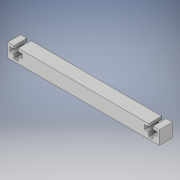
# Autodesk Inventor part: horzntalconnection
Saved by Autodesk Inventor 2017 (Build 210142000, 142)
## iProperties
Created: 2017-11-22
Part Number: horzntalconnection
Material: Generic
Document SubType Name: Modeling
Designer: build
Density: 1 g/cm^3
Appearance: Default
Author: build
Autodesk Inventor part; units mm, degrees
ref_plane "YZ Plane" through (0, 0, 0) normal (1, 0, 0) x (0, 1, 0)
ref_plane "XZ Plane" through (0, 0, 0) normal (0, 1, 0) x (-1, 0, 0)
ref_plane "XY Plane" through (0, 0, 0) normal (0, 0, 1) x (1, 0, 0)
sketch "Sketch1" plane through (0, 0, 0) normal (1, 0, 0) x (0, 1, 0)
  line L0 (0, 0) -> (16.383, 0)
  line L1 (16.383, 0) -> (16.383, -15.875)
  line L2 (16.383, -15.875) -> (0, -15.875)
  line L3 (0, -15.875) -> (0, 0)
  dimension "d0" = 16.383
  dimension "d1" = 15.875
  constraints: 8 end point, 2 parallel, 1 horizontal, 1 perpendicular
  measures "d0" distance of L0.start L0.end
  measures "d1" distance of L0.end L1.end
extrude "Extrusion1" add sketch "Sketch1" along normal blind 184.15
sketch "Sketch2" plane through (0, 0, -15.875) normal (0, 0, -1) x (-1, 0, 0)
  line L0 (-184.15, 16.383) -> (-184.15, 0) projected
  line L1 (-184.15, 16.383) -> (-176.53, 16.383)
  line L2 (0, 16.383) -> (-184.15, 16.383) projected
  line L3 (-176.53, 16.383) -> (-176.53, 13.081)
  line L4 (-176.53, 13.081) -> (-181.61, 13.081)
  line L5 (-181.61, 13.081) -> (-181.61, 8.001)
  line L6 (-181.61, 8.001) -> (-176.53, 8.001)
  line L7 (-176.53, 8.001) -> (-176.53, 2.921)
  line L8 (-176.53, 2.921) -> (-171.45, 2.921)
  line L9 (-171.45, 2.921) -> (-171.45, 8.001)
  line L10 (-171.45, 8.001) -> (-166.37, 8.001)
  line L11 (-166.37, 8.001) -> (-166.37, 13.081)
  line L12 (-166.37, 13.081) -> (-171.45, 13.081)
  line L13 (-171.45, 16.383) -> (-171.45, 13.081)
  line L14 (0, 16.383) -> (-7.62, 16.383)
  line L15 (-7.62, 16.383) -> (-7.62, 13.081)
  line L16 (-7.62, 13.081) -> (-2.54, 13.081)
  line L17 (-2.54, 13.081) -> (-2.54, 8.001)
  line L18 (-2.54, 8.001) -> (-7.62, 8.001)
  line L19 (-7.62, 8.001) -> (-7.62, 2.921)
  line L20 (-7.62, 2.921) -> (-12.7, 2.921)
  line L21 (-12.7, 2.921) -> (-12.7, 8.001)
  line L22 (-12.7, 8.001) -> (-17.78, 8.001)
  line L23 (-17.78, 8.001) -> (-17.78, 13.081)
  line L24 (-17.78, 13.081) -> (-12.7, 13.081)
  line L25 (-12.7, 13.081) -> (-12.7, 16.383)
  point P0 (0, 0)
  dimension "d4" = 7.62
  dimension "d5" = 3.302
  dimension "d6" = 5.08
  dimension "d7" = 5.08
  dimension "d8" = 5.08
  dimension "d9" = 5.08
  dimension "d10" = 5.08
  dimension "d11" = 7.62
  dimension "d12" = 3.302
  dimension "d13" = 5.08
  dimension "d14" = 5.08
  dimension "d15" = 5.08
  constraints: 48 end point, 14 perpendicular, 13 point on line, 3 vertical, 1 horizontal, 1 parallel
  measures "d4" distance of L0.start L1.end
  measures "d5" distance of L1.end L3.end
  measures "d6" distance of L3.end L4.end
  measures "d7" distance of L4.end L5.end
  measures "d8" distance of L6.end L7.end
  measures "d9" distance of L7.end L8.end
  measures "d10" distance of L9.end L10.end
  measures "d11" distance of L2.start L14.end
  measures "d12" distance of L14.end L15.end
  measures "d13" distance of L15.end L16.end
  measures "d14" distance of L19.end L20.end
  measures "d15" distance of L21.end L22.end
extrude "Extrusion2" cut sketch "Sketch2" against normal blind 184.15
shell "Shell1" thickness 1.778 removed faces 0
body "Solid1"
